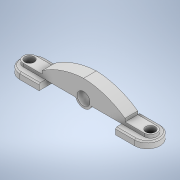
# Autodesk Inventor part: camfer,fillet dan holes
Saved by Autodesk Inventor 2021 (Build 250183000, 183)
## iProperties
Created: 2022-03-13
Part Number: camfer,fillet dan holes
Material: Generic
Document SubType Name: Modeling
Designer: User
Density: 1 g/cm^3
Appearance: Default
Author: User
Autodesk Inventor part; units mm, degrees
ref_plane "YZ Plane" through (0, 0, 0) normal (1, 0, 0) x (0, 1, 0)
ref_plane "XZ Plane" through (0, 0, 0) normal (0, 1, 0) x (-1, 0, 0)
sketch "Sketch1" plane through (0, 0, 0) normal (0, 1, 0) x (-1, 0, 0)
  line L0 (11, -8) -> (6, -8)
  line L1 (6, -8) -> (6, -4)
  line L2 (6, -4) -> (11, -4)
  line L3 (11, -4) -> (11, -8)
  line L4 (-6, -4) -> (-11, -4)
  line L5 (-11, -4) -> (-11, -8)
  line L6 (-11, -8) -> (-6, -8)
  line L7 (-6, -8) -> (-6, -4)
  point P0 (0, 0)
  dimension "d0" = 5
  dimension "d1" = 4
  dimension "d2" = 6
  dimension "d3" = 4
  dimension "d4" = 5
  dimension "d5" = 4
  dimension "d6" = 6
  dimension "d7" = 4
  constraints: 16 end point, 4 parallel, 2 horizontal, 2 perpendicular
  measures "d0" distance of L1.end L2.end
  measures "d1" distance of L0.end L1.end
  measures "d2" distance from line of L1 point (0, 0)
  measures "d3" distance from line of L2 point (0, 0)
  measures "d4" distance of L6.end L5.end
  measures "d5" distance of L5.end L4.end
  measures "d6" distance from line of L7 point (0, 0)
  measures "d7" distance from line of L4 point (0, 0)
extrude "Extrusion1" add sketch "Sketch1" along normal blind 1
ref_plane "Work Plane1" through (0, 0, -5) normal (0, 0, 1) x (1, 0, 0)
sketch "Sketch3" plane through (0, 0, -5) normal (0, 0, 1) x (1, 0, 0)
  line L0 (11, 1) -> (11, 0) projected
  line L1 (11, 0) -> (6, 0) projected
  line L2 (6, 0) -> (6, 1) projected
  line L3 (6, 1) -> (11, 1) projected
  line L4 (-6, 1) -> (-6, 0) projected
  line L5 (-6, 0) -> (-11, 0) projected
  line L6 (-11, 0) -> (-11, 1) projected
  line L7 (-11, 1) -> (-6, 1) projected
  line L8 (-6, 1) -> (-11, 1) projected
  line L9 (6.5, 1) -> (6.5, 2)
  line L10 (-6.5, 2) -> (-6.5, 1)
  arc A0 (-1.2346, 1) -> (1.2346, 1) centre (0, 1.407) ccw
  line L11 (-6.5, 1) -> (-1.2346, 1)
  line L12 (1.2346, 1) -> (6.5, 1)
  arc A1 (0, 4.1975) -> (-6.5, 2) centre (0.6617, -8.4719) ccw
  arc A2 (6.5, 2) -> (0, 4.1975) centre (-0.3857, -7.6555) ccw
  line L13 (6.5, 2) -> (6, 2)
  line L14 (-6, 2) -> (-6.5, 2)
  point P0 (0, 0)
  point P1 (6, 1)
  dimension "d11" = 13
  dimension "d12" = 1
  dimension "d13" = 6.5
  dimension "d14" = 2.6
  constraints: 12 end point, 6 point on circle, 5 parallel, 3 centre point, 3 point on line, 2 horizontal, 2 perpendicular
  measures "d11" distance of L10.start L9.end
  measures "d12" distance of L9.end L9.start
  measures "d13" distance from line of L10 point (0, 0)
  measures "d14" diameter of A0
extrude "Extrusion2" add sketch "Sketch3" against normal blind 2 contours L3 L12 A0 L11 L7 L10 A1 A2 L9
sketch "Sketch4" plane through (0, 1, 0) normal (0, 1, 0) x (1, 0, 0)
  line L0 (0, 7) -> (-6.5, 7) projected
  line L1 (-6.5, 7) -> (-9.5, 7)
  line L2 (-9.5, 7) -> (-9.5, 5)
  line L3 (-9.5, 5) -> (-6.5, 5)
  line L4 (-6.5, 5) -> (-6.5, 7)
  arc A0 (-9.5, 7) -> (-9.5, 5) centre (-9.5, 6) ccw
  line L5 (6.5, 5) -> (6, 5) projected
  line L6 (6.5, 5) -> (9.5, 5)
  line L7 (9.5, 5) -> (9.5, 7)
  line L8 (9.5, 7) -> (6.5, 7)
  line L9 (6.5, 7) -> (6.5, 5)
  arc A1 (9.5, 5) -> (9.5, 7) centre (9.5, 6) ccw
  point P0 (0, 0)
  dimension "d17" = 3
  dimension "d18" = 2
  dimension "d19" = 1
  dimension "d20" = 3
  dimension "d21" = 2
  dimension "d22" = 1
  constraints: 16 end point, 4 parallel, 4 point on circle, 2 centre point, 2 horizontal, 2 perpendicular
  measures "d17" distance of L3.end L2.end
  measures "d18" distance of L2.end L1.end
  measures "d19" radius of A0
  measures "d20" distance of L8.end L7.end
  measures "d21" distance of L7.end L6.end
  measures "d22" radius of A1
extrude "Extrusion3" add sketch "Sketch4" along normal blind 0.5
sketch "Sketch5" plane through (0, 1.5, 0) normal (0, 1, 0) x (1, 0, 0)
  arc A0 (-9.5, 7) -> (-9.5, 5) centre (-9.5, 6) ccw projected
  point P0 (0, 0)
  constraints: 1 coincident
hole "Hole1" at (-9.5, 1.5, -6) direction (0, -1, 0) diameter 1 end through all counterbore diameter 1.5 counterbore depth 1
sketch "Sketch6" plane through (0, 1.5, 0) normal (0, 1, 0) x (1, 0, 0)
  arc A0 (9.5, 5) -> (9.5, 7) centre (9.5, 6) ccw projected
  point P0 (0, 0)
  constraints: 1 coincident
hole "Hole2" at (9.5, 1.5, -6) direction (0, -1, 0) diameter 1 end through all counterbore diameter 1.5 counterbore depth 1
sketch "Sketch7" plane through (0, 0, -5) normal (0, 0, 1) x (1, 0, 0)
  arc A0 (-1.2346, 1) -> (1.2346, 1) centre (0, 1.407) ccw projected
  point P0 (0, 0)
  constraints: 1 coincident
hole "Hole3" at (0, 1.407, -5) direction (0, 0, -1) diameter 2 end through all
fillet "Fillet1" radius 2 4 edges at (-11, 0.5, -4) (-11, 0.5, -8) (11, 0.5, -8) (11, 0.5, -4)
chamfer "Chamfer1" distance 0.2 angle 45 3 edges at (-7.5003, 1, -4) (-10.4144, 1, -4.5856) (-7.5003, 1, -8)
chamfer "Chamfer2" distance 0.2 angle 45 3 edges at (7.5002, 1, -4) (10.4144, 1, -7.4144) (7.5002, 1, -8)
body "Solid1"
